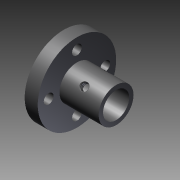
# Autodesk Inventor part: BTHR12-MB_b
Saved by Autodesk Inventor 2011 SP1 (Build 150282100, 282)
## iProperties
Created: 2016-04-10
Part Number: BTHR12-MB_b
Catalog Web Link: www.cadenas.de
Description: STHRB, STHR, SSTHR, ATHR, BTHR_b-Shaft Supports - Bracket Shaped - Standard Drilled Mounting Hole Type - Round Flange
Vendor: MISUMI
Document SubType Name: Modeling
Designer: psAdmin
Manufacturer: MISUMI
Mass: 6.59623 g
Surface Area: 45.1421 cm^2
Volume: 6.59623 cm^3
Density: 1 g/cm^3
Category: PARTsolutions
Company: MISUMI
Title: BTHR12-MB
Author: Cadenas PARTsolutions
Comments: Shaft Supports - Bracket Shaped - Standard Drilled Mounting Hole Type - Round Flange
PSOL_IDENT_0: {$CADENAS_DATA\23d-libs\misumi\metric\02_shaft_supports\ssthr\ssthr_body.prj},200 {VTYP=3D},{NB=BTHR
PSOL_IDENT_1: 12-MB_b},{LINA=BTHR12-MB},{NN=STHRB, STHR, SSTHR, ATHR, BTHR_b},{DATE=07.10.2015 06:02:59},{GEOMDATE=
PSOL_IDENT_2: 06.10.2015 08:50:00},{VERSION=},{LINEID=70},{LINESUBID=-1},{WBVAR=MAT,ST,M,ALT}  {NB=BTHR12-MB_b},{L
PSOL_IDENT_3: INA=BTHR12-MB},{KT=DUMMY},{PN=BTHR12-MB},{TS=1},{TSALG= '1', 'Drilled Mounting Hole', '2', 'Tapped M
PSOL_IDENT_4: ounting Hole' },{TYPE=BTHR},{MAT=AA},{MATA= '1018', 'SS400 Equivalent', '304', 'SUS304', 'AA'  , 'Al
PSOL_IDENT_5: uminum Alloy' },{MALG='M4'},{ST=BA},{ST0= 'CA', 'Clear Anodizing', 'BA', 'Black Anodizing' },{D=12},
PSOL_IDENT_6: {THMD11='M4'},{THMD13='M4'},{THMD12='M4'},{DTOL=+0.018/0},{DX=12},{N=2.0},{L=24},{D1=16},{H=36},{T=6
PSOL_IDENT_7: .0},{LL=15},{M=M4},{THMD=4},{THMD1=M4},{THMD2=M4},{P=26},{K=28},{W=20},{P1=26},{F=0},{DD1=4.5},{DD11=
PSOL_IDENT_8: 4.5},{DD12=4.5},{M1=M4},{M11=4},{ALT=MB},{ALTPN=-MB},{BM=4.0},{BL=3.0}
NN: STHRB, STHR, SSTHR, ATHR, BTHR_b
NT: Shaft Supports - Bracket Shaped - Standard Drilled Mounting Hole Type - Round Flange
NB: BTHR12-MB_b
NBSYN: $PN._b
LINA: BTHR12-MB
PN: BTHR12-MB
MAT: Aluminum Alloy
ST: Black Anodizing
D: 12
DTOL: +0.018/0
N: 2.0
L: 24
D1: 16
H: 36
T: 6.0
LL: 15
M: M4
P: 26
DD1: 4.5
ALT: with MB (Hex Socket Set Screw Included)
SUPPLIER: MISUMI
ARTICLENO: BTHR12-MB_b
BOMINFO: BTHR12-MB
CREATOR: CADENAS GmbH
Autodesk Inventor part; units mm, degrees
sketch "Sketch_1" plane through (0, 0, 0) normal (0, 0, 1) x (1, 0, 0)
  line L0 (24, 0) -> (0, 0)
  line L1 (0, 18) -> (0, 6)
  line L2 (0, 6) -> (24, 6)
  line L3 (24, 6) -> (24, 8)
  line L4 (24, 8) -> (6, 8)
  line L5 (6, 8) -> (6, 18)
  line L6 (6, 18) -> (0, 18)
  constraints: 14 end point
revolve "Revolution1" add sketch "Sketch_1" angle 360 about axis through (24, 0, 0) along (1, 0, 0)
sketch "Sketch_3" plane through (0, 0, 0) normal (0, -0.7071, 0.7071) x (1, 0, 0)
  line L0 (15, 5.5) -> (15, 8)
  line L1 (15, 8) -> (17, 8)
  line L2 (17, 8) -> (16.621, 7.621)
  line L3 (16.621, 7.621) -> (16.621, 5.5)
  line L4 (16.621, 5.5) -> (15, 5.5)
  line L5 (15, 5.5) -> (15, 8)
  constraints: 12 end point
revolve "Revolution2" cut sketch "Sketch_3" angle 360 about axis through (15, 3.8891, 3.8891) along (0, -0.7071, -0.7071)
thread "Thread1" size "M4x0.7" class "6H" standard "ISO Metric profile" length 2.121
sketch "Sketch3" plane through (6, 0, 0) normal (1, 0, 0) x (0, 0, -1)
  point P0 (0, 13)
hole "Hole1" at (6, 13, 0) direction (-1, 0, 0) diameter 4.5 depth 6
sketch "Sketch4" plane through (6, 0, 0) normal (1, 0, 0) x (0, 0, -1)
  point P0 (0, -13)
hole "Hole2" at (6, -13, 0) direction (-1, 0, 0) diameter 4.5 depth 6
sketch "Sketch5" plane through (6, 0, 0) normal (1, 0, 0) x (0, 0, -1)
  point P0 (-13, 0)
hole "Hole3" at (6, 0, 13) direction (-1, 0, 0) diameter 4.5 depth 6
sketch "Sketch6" plane through (6, 0, 0) normal (1, 0, 0) x (0, 0, -1)
  point P0 (13, 0)
hole "Hole4" at (6, 0, -13) direction (-1, 0, 0) diameter 4.5 depth 6
sketch "Sketch_2" plane through (0, 0, 0) normal (0, -0.7071, -0.7071) x (1, 0, 0)
  line L0 (15, 5.5) -> (15, 8)
  line L1 (15, 8) -> (17, 8)
  line L2 (17, 8) -> (16.621, 7.621)
  line L3 (16.621, 7.621) -> (16.621, 5.5)
  line L4 (16.621, 5.5) -> (15, 5.5)
  line L5 (15, 5.5) -> (15, 8)
  constraints: 12 end point
revolve "Revolution3" cut sketch "Sketch_2" angle 360 about axis through (15, -3.8891, 3.8891) along (0, 0.7071, -0.7071)
thread "Thread2" size "M4x0.7" class "6H" standard "ISO Metric profile" length 2.121
ref_plane "to_screw1_XY" through (15, 4.2426, 4.2426) normal (0, 0.7071, 0.7071) x (1, 0, 0)
ref_plane "to_screw1_YZ" through (15, 4.2426, 4.2426) normal (1, 0, 0) x (0, 0.7071, -0.7071)
ref_plane "to_screw1_ZX" through (15, 4.2426, 4.2426) normal (0, 0.7071, -0.7071) x (0, 0.7071, 0.7071)
ref_plane "to_screw2_XY" through (15, -4.2426, 4.2426) normal (0, -0.7071, 0.7071) x (1, 0, 0)
ref_plane "to_screw2_YZ" through (15, -4.2426, 4.2426) normal (1, 0, 0) x (0, 0.7071, 0.7071)
ref_plane "to_screw2_ZX" through (15, -4.2426, 4.2426) normal (0, 0.7071, 0.7071) x (0, -0.7071, 0.7071)
body "Solid1"
